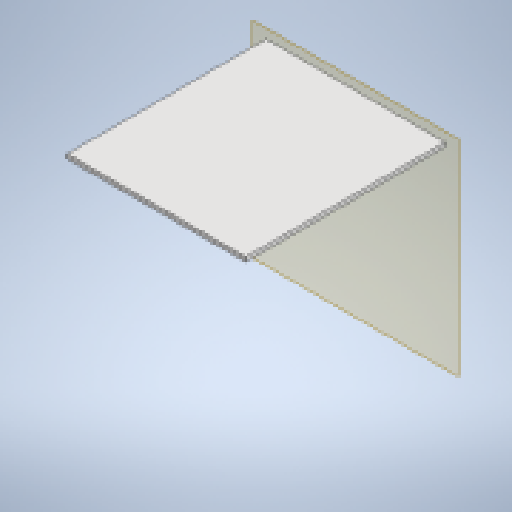
# Autodesk Inventor part: AcrilicoY
Saved by Autodesk Inventor 2024 (Build 280153000, 153)
## iProperties
Created: 2023-06-26
Part Number: AcrilicoY
Material: Genérico
Document SubType Name: Modeling
Designer: Personal
Density: 1 g/cm^3
Appearance: Valor por defecto
Author: Personal
Autodesk Inventor part; units mm, degrees
ref_plane "YZ Plane" through (0, 0, 0) normal (1, 0, 0) x (0, 1, 0)
ref_plane "XZ Plane" through (0, 0, 0) normal (0, 1, 0) x (-1, 0, 0)
ref_plane "XY Plane" through (0, 0, 0) normal (0, 0, 1) x (1, 0, 0)
ref_plane "Plano de trabajo1" through (0, 0, 0) normal (0, 0, 1) x (1, 0, 0)
sketch "Boceto1" plane through (0, 0, 0) normal (0, 0, 1) x (1, 0, 0)
  line L0 (97.5, 97.5) -> (-97.5, 97.5) construction
  line L1 (93.1, -97.5) -> (93.1, 97.5) construction
  line L2 (-93.1, -97.5) -> (-93.1, 97.5) construction
  line L3 (93.1, 93.1) -> (-93.1, 93.1)
  line L4 (-93.1, 93.1) -> (-93.1, 97.5)
  line L5 (-93.1, 97.5) -> (93.1, 97.5)
  line L6 (93.1, 97.5) -> (93.1, 93.1)
  point P0 (0, 0)
  dimension "d0" = 4.4
  constraints: 8 end point, 2 parallel, 1 horizontal, 1 perpendicular, 1 point on line
  measures "d0" distance between parallel lines of L0 L3
extrude "Extrusión1" add sketch "Boceto1" along normal blind 207.6
